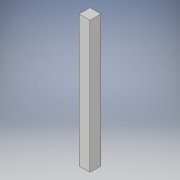
# Autodesk Inventor part: rev1 base short wall v stud
Saved by Autodesk Inventor 2017 (Build 210142000, 142)
## iProperties
Created: 2019-05-04
Part Number: rev1 base short wall v stud
Material: Generic
Document SubType Name: Modeling
Designer: Roman
Density: 1 g/cm^3
Appearance: Default
Author: Roman
Autodesk Inventor part; units mm, degrees
ref_plane "YZ Plane" through (0, 0, 0) normal (1, 0, 0) x (0, 1, 0)
ref_plane "XZ Plane" through (0, 0, 0) normal (0, 1, 0) x (-1, 0, 0)
ref_plane "XY Plane" through (0, 0, 0) normal (0, 0, 1) x (1, 0, 0)
sketch "Sketch1" plane through (0, 0, 0) normal (1, 0, 0) x (0, 1, 0)
  line L0 (0, 0) -> (-609.6, 0)
  line L1 (-609.6, 0) -> (-609.6, -50.8)
  line L2 (-609.6, -50.8) -> (0, -50.8)
  line L3 (0, -50.8) -> (0, 0)
  dimension "d0" = 609.6
  dimension "d1" = 50.8
  constraints: 8 end point, 2 parallel, 1 horizontal, 1 perpendicular
  measures "d0" distance of L2.end L1.end
  measures "d1" distance of L1.end L0.end
extrude "Extrusion1" add sketch "Sketch1" along normal blind 50.8
body "Solid1"
